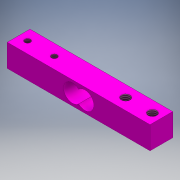
# Autodesk Inventor part: celda de carga
Saved by Autodesk Inventor 2018 (Build 220112000, 112)
## iProperties
Created: 2019-05-16
Part Number: celda de carga
Material: Generic
Document SubType Name: Modeling
Designer: JLVega003
Density: 1 g/cm^3
Appearance: Magenta
Author: JLVega003
Autodesk Inventor part; units mm, degrees
ref_plane "YZ Plane" through (0, 0, 0) normal (1, 0, 0) x (0, 1, 0)
ref_plane "XZ Plane" through (0, 0, 0) normal (0, 1, 0) x (-1, 0, 0)
ref_plane "XY Plane" through (0, 0, 0) normal (0, 0, 1) x (1, 0, 0)
sketch "Sketch1" plane through (0, 0, 0) normal (0, 0, 1) x (1, 0, 0)
  line L0 (-40, -6.35) -> (40, -6.35)
  line L1 (40, -6.35) -> (40, 6.35)
  line L2 (40, 6.35) -> (-40, 6.35)
  line L3 (-40, 6.35) -> (-40, -6.35)
  line L4 (-40, -6.35) -> (40, 6.35) construction
  line L5 (40, -6.35) -> (-40, 6.35) construction
  point P0 (0, 0)
  dimension "d0" = 80
  dimension "d1" = 12.7
  constraints: 12 end point, 2 midpoint, 2 parallel, 1 horizontal, 1 perpendicular
  measures "d0" distance of L2.end L1.end
  measures "d1" distance between parallel lines of L0 L2
extrude "Extrusion1" add sketch "Sketch1" along normal mid plane 12.7
sketch "Sketch2" plane through (0, 0, 6.35) normal (0, 0, 1) x (1, 0, 0)
  line L0 (-20, 0) -> (20, 0)
  line L1 (20, 0) -> (35, 0)
  line L2 (-20, 0) -> (-35, 0)
  point P0 (0, 0)
  point P1 (0, 0)
  dimension "d4" = 40
  dimension "d5" = 15
  dimension "d6" = 15
  constraints: 6 end point, 5 coincident, 2 horizontal, 1 midpoint, 1 point on line
  measures "d4" distance of L0.end L0.start
  measures "d5" distance of L0.start L2.end
  measures "d6" distance of L1.end point (20, 0)
hole "Hole1" at (-35, 0, 6.35) at (-20, 0, 6.35) direction (0, 0, -1) diameter 3.242 end through all thread size "M4x0.7" class "6H" standard "ISO Metric profile"
hole "Hole2" at (20, 0, 6.35) at (35, 0, 6.35) direction (0, 0, -1) diameter 4.917 end through all thread size "M6x1" class "6H" standard "ISO Metric profile"
sketch "Sketch3" plane through (-40, 6.35, 6.35) normal (0, 1, 0) x (1, 0, 0)
  line L0 (36.5, 6.35) -> (43.5, 6.35)
  point P0 (40, 6.35)
  point P1 (40, 6.35)
  dimension "d28" = 7
  constraints: 3 coincident, 2 end point, 1 horizontal, 1 midpoint
  measures "d28" distance of L0.start L0.end
hole "Hole3" at (-3.5, 6.35, 0) at (3.5, 6.35, 0) direction (0, -1, 0) diameter 10 end through all
body "Solid1"
